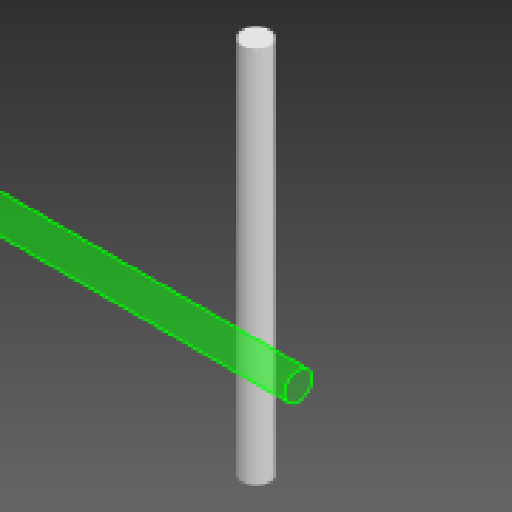
# Autodesk Inventor part: axis
Saved by Autodesk Inventor 2023 (Build 270158000, 158)
## iProperties
Created: 2025-06-01
Part Number: axis
Material: Типовые
Document SubType Name: Modeling
Designer: daa
Density: 1 g/cm^3
Appearance: По умолчанию
Author: daa
Autodesk Inventor part; units mm, degrees
ref_plane "YZ Plane" through (0, 0, 0) normal (1, 0, 0) x (0, 1, 0)
ref_plane "XZ Plane" through (0, 0, 0) normal (0, 1, 0) x (-1, 0, 0)
ref_plane "XY Plane" through (0, 0, 0) normal (0, 0, 1) x (1, 0, 0)
sketch "Эскиз1" plane through (0, 0, 0) normal (0, 1, 0) x (-1, 0, 0)
  circle A0 centre (0, 0) radius 2
  dimension "d0" = 4
  constraints: 1 centre point, 1 coincident
  measures "d0" diameter of A0
extrude "Выдавливание1" add sketch "Эскиз1" along normal blind 55
